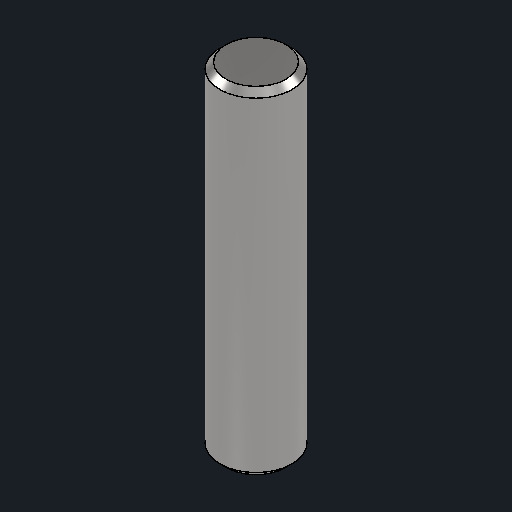
# Autodesk Inventor part: 3x30 Pin
Saved by Autodesk Inventor 2026.1 (Build 301233020, 233B)
## iProperties
Created: 2025-05-24
Part Number: 3x30 Pin
Material: Stainless Steel, 440C
Document SubType Name: Modeling
Designer: Joshua Eah
Density: 7.75 g/cm^3
Appearance: Semi-Polished
Author: Joshua Eah
Autodesk Inventor part; units mm, degrees
ref_plane "YZ Plane" through (0, 0, 0) normal (1, 0, 0) x (0, 1, 0)
ref_plane "XZ Plane" through (0, 0, 0) normal (0, 1, 0) x (-1, 0, 0)
ref_plane "XY Plane" through (0, 0, 0) normal (0, 0, 1) x (1, 0, 0)
sketch "Sketch1" plane through (0, 0, 0) normal (0, 1, 0) x (-1, 0, 0)
  circle A0 centre (0, 0) radius 1.5
  dimension "d0" = 3
  constraints: 1 centre point, 1 coincident
  measures "d0" diameter of A0
extrude "Extrusion1" add sketch "Sketch1" along normal blind 14
chamfer "Chamfer1" distance 0.25 angle 45 2 edges at (1.5, 14, 0) (1.5, 0, 0)
body "Solid1"
